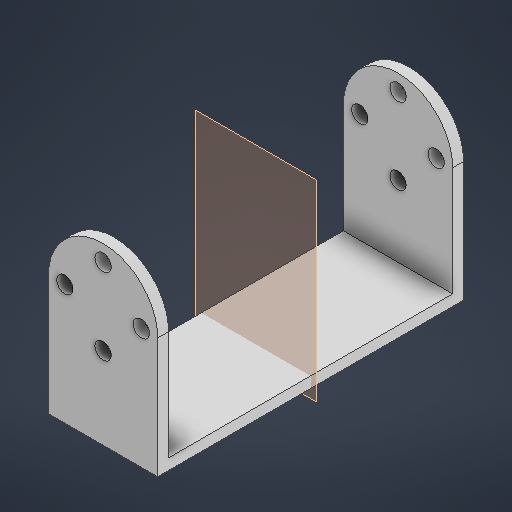
# Autodesk Inventor part: Bracket
Saved by Autodesk Inventor 2026 (Build 300175050, 175E)
## iProperties
Created: 2025-08-11
Part Number: Bracket
Material: Generic
Document SubType Name: Modeling
Designer: sidsi
Density: 1 g/cm^3
Appearance: Default
Author: sidsi
Autodesk Inventor part; units mm, degrees
ref_plane "YZ Plane" through (0, 0, 0) normal (1, 0, 0) x (0, 1, 0)
ref_plane "XZ Plane" through (0, 0, 0) normal (0, 1, 0) x (-1, 0, 0)
ref_plane "Work Plane1" through (-10, 0, 28) normal (0, -1, 0) x (1, 0, 0)
sketch "Sketch3" plane through (-10, 0, 28) normal (0, -1, 0) x (1, 0, 0)
  line L0 (-10, -28) -> (10, -28)
  line L1 (10, -28) -> (10, 28)
  line L2 (10, 28) -> (-10, 28)
  line L3 (-10, 28) -> (-10, -28)
  line L4 (10, 28) -> (-10, 28)
  line L5 (-10, 28) -> (-10, 31)
  line L6 (-10, 31) -> (10, 31)
  line L7 (10, 31) -> (10, 28)
  line L8 (10, -28) -> (-10, -28)
  line L9 (-10, -28) -> (-10, -31)
  line L10 (-10, -31) -> (10, -31)
  line L11 (10, -31) -> (10, -28)
  line L12 (10, 28) -> (5, 28)
  line L13 (5, 28) -> (5, -28)
  line L14 (-10, 28) -> (-5, 28)
  line L15 (-5, 28) -> (-5, -28)
  line L16 (5, 28) -> (5, 14)
  circle A0 centre (5, 14) radius 1.5
  line L17 (5, 14) -> (5, 4)
  circle A1 centre (5, 4) radius 1.5
  line L18 (10, 28) -> (10, 0)
  line L19 (10, 0) -> (-10, 0)
  circle A2 centre (0, 0) radius 3
  line L20 (0, 28) -> (0, -28)
  circle A3 centre (-5, 4) radius 1.5
  circle A4 centre (-5, 14) radius 1.5
  circle A5 centre (5, -14) radius 1.5
  circle A6 centre (5, -4) radius 1.5
  circle A7 centre (-5, -4) radius 1.5
  circle A8 centre (-5, -14) radius 1.5
  point P0 (10, -28)
  point P1 (-10, 28)
  dimension "d13" = 20
  dimension "d14" = 56
  dimension "d15" = 3
  dimension "d16" = 3
  dimension "d17" = 5
  dimension "d18" = 5
  dimension "d19" = 14
  dimension "d20" = 3
  dimension "d21" = 10
  dimension "d22" = 3
  dimension "d23" = 6
  constraints: 42 end point, 9 centre point, 7 point on line, 6 parallel, 6 symmetric about line, 5 midpoint, 5 perpendicular, 3 horizontal, 2 coincident, 6 other
  measures "d13" distance of L2.end L1.end
  measures "d14" distance of L1.end L0.end
  measures "d15" distance of L4.end L5.end
  measures "d16" distance of L9.end L8.end
  measures "d17" distance of L1.end L12.end
  measures "d18" distance of L4.end L14.end
  measures "d19" distance of L12.end L16.end
  measures "d20" diameter of A0
  measures "d21" distance of L17.start L17.end
  measures "d22" diameter of A1
  measures "d23" diameter of A2
extrude "Extrusion2" add sketch "Sketch3" along normal blind 2 contours L3 L19 L15 A7 A8 L0 | L15 A8 A7 L19 A2 L20 L0 | L3 L2 L15 A4 A3 L19 | L20 A2 L19 L13 A6 A5 L0 | A8 L15 | L15 A8 | L15 A3 A4 L2 L20 A2 L19 | L13 A5 A6 L19 L1 L0 | L20 L19 A2 | A2 L19 L20 | A3 L15 | L15 A3 | A7 L15 | L15 A7 | A2 L20 L19 | A5 L13 | L13 A5 | A2 L20 L2 L13 A0 A1 L19 | L19 L20 A2 | A4 L15 | L15 A4 | L19 L13 A1 A0 L2 L1 | A6 L13 | L13 A6 | A1 L13 | L13 A1 | A0 L13 | L13 A0
sketch "Sketch5" plane through (-10, 0, 28) normal (0, 1, 0) x (1, 0, 0)
  line L0 (-10, -28) -> (-10, 28) projected
  line L1 (10, 28) -> (-10, 28)
  line L2 (-10, 28) -> (-10, 26)
  line L3 (-10, 26) -> (10, 26)
  line L4 (10, 26) -> (10, 28)
  line L5 (10, 28) -> (10, -28) projected
  line L6 (10, -28) -> (-10, -28)
  line L7 (-10, -28) -> (-10, -26)
  line L8 (-10, -26) -> (10, -26)
  line L9 (10, -26) -> (10, -28)
  dimension "d26" = 2
  dimension "d27" = 2
  constraints: 16 end point, 4 parallel, 2 horizontal, 2 perpendicular, 2 point on line
  measures "d26" distance of L2.end L1.end
  measures "d27" distance of L6.end L7.end
extrude "Extrusion3" add sketch "Sketch5" along normal blind 20 contours L0 L1 L4 L3
sketch "Sketch6" plane through (0, -2, 0) normal (0, 0, -1) x (-1, 0, 0)
  line L0 (0, 22) -> (20, 22) projected
  circle A0 centre (10, 22) radius 10
  point P0 (0, 2)
  constraints: 1 midpoint, 3 other
extrude "Extrusion4" add sketch "Sketch6" against normal up to surface (2 mm away) contours A0 L0 picked at (13.2365, 22.7977)
sketch "Sketch7" plane through (0, -2, 0) normal (0, 0, -1) x (-1, 0, 0)
  arc A0 (20, 22) -> (0, 22) centre (10, 22) ccw projected
  circle A1 centre (10, 22) radius 7
  circle A2 centre (10, 15) radius 1.5
  circle A3 centre (3, 22) radius 1.5
  circle A4 centre (10, 29) radius 1.5
  circle A5 centre (17, 22) radius 1.5
  point P0 (0, 2)
  dimension "d32" = 14
  dimension "d33" = 3
  dimension "d34" = 3
  dimension "d35" = 3
  dimension "d36" = 3
  constraints: 5 centre point, 4 point on circle, 1 coincident
  measures "d32" diameter of A1
  measures "d33" diameter of A2
  measures "d34" diameter of A3
  measures "d35" diameter of A4
  measures "d36" diameter of A5
extrude "Extrusion5" cut sketch "Sketch7" against normal blind 10 contours A1 A5 | A1 A5 | A4 A1 | A1 A4 | A2 A1 | A1 A2 | A3 A1 | A1 A3
ref_plane "Work Plane2" through (-20, 0, 28) normal (0, 0, 1) x (1, 0, 0)
mirror "Mirror1" about plane through (-20, 0, 28) normal (0, 0, 1) of "Extrusion4", "Extrusion5", "Extrusion3"
body "Solid1"
